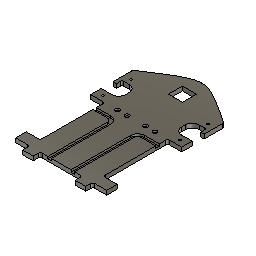
2023_2024_3DP_07.03_Robot_follow_line_v3 (Autodesk Fusion 360 design; units mm, degrees)
Autodesk Fusion 360 part; units mm, degrees
note: some values were not read from the file. Set by a fixed rule: the direction of a hole.
sketch "Sketch1" plane through (0, 0, 0) normal (0, 0, 1) x (1, 0, 0)
  line L0 (-65, -210) -> (-48, -210)
  line L1 (-45, -213) -> (-45, -220)
  line L2 (-45, -220) -> (-30, -220)
  line L3 (-30, -220) -> (-30, -213)
  line L4 (-27, -210) -> (0, -210)
  arc A0 (-45, -213) -> (-48, -210) centre (-48, -213) ccw
  arc A1 (-27, -210) -> (-30, -213) centre (-27, -213) ccw
  line L5 (-65, -210) -> (-65, -195)
  line L6 (-65, -195) -> (-48, -195)
  line L7 (-45, -192) -> (-45, -106)
  line L8 (-48, -103) -> (-65, -103)
  line L9 (-65, -103) -> (-65, -88)
  line L10 (-65, -88) -> (-50, -88)
  line L11 (-40, -78) -> (-40, -73)
  line L12 (-65, -63) -> (-65, -44.6163)
  arc A2 (-50, -88) -> (-40, -78) centre (-50, -78) ccw
  arc A3 (-40, -73) -> (-50, -63) centre (-50, -73) ccw
  arc A4 (-48, -195) -> (-45, -192) centre (-48, -192) ccw
  arc A5 (-45, -106) -> (-48, -103) centre (-48, -106) ccw
  line L13 (-65, -63) -> (-65, -71)
  line L14 (-65, -71) -> (-60, -71)
  line L15 (-60, -71) -> (-60, -65)
  line L16 (-58, -63) -> (-50, -63)
  arc A6 (-58, -63) -> (-60, -65) centre (-58, -65) ccw
  line L17 (-63.6502, -42.1109) -> (-56.6488, -37.4994)
  arc A7 (-63.6502, -42.1109) -> (-65, -44.6163) centre (-62, -44.6163) ccw
  line L18 (0, 0) -> (0, -252.3978) construction
  spline S0 degree 2 poles (-56.6488, -37.4994) (-14.1632, -9.3755) (0, -9.5) knots 0 0 0 6.369294 6.369294 6.369294 weights 1 1.414179 1
  line L19 (-10, -27) -> (0, -27)
  line L20 (0, -47) -> (-10, -47)
  line L21 (-10, -47) -> (-10, -27)
  circle A8 centre (-13, -103) radius 3
  circle A9 centre (-27, -103) radius 3
  line L22 (-13, -103) -> (-27, -103)
  line L23 (45, -220) -> (30, -220)
  line L24 (63.6502, -42.1109) -> (56.6488, -37.4994)
  line L25 (65, -210) -> (48, -210)
  line L26 (45, -192) -> (45, -106)
  line L27 (58, -63) -> (50, -63)
  line L28 (65, -88) -> (50, -88)
  line L29 (0, -47) -> (10, -47)
  line L30 (65, -71) -> (60, -71)
  arc A10 (48, -210) -> (45, -213) centre (48, -213) ccw
  line L31 (48, -103) -> (65, -103)
  arc A11 (50, -63) -> (40, -73) centre (50, -73) ccw
  line L32 (10, -27) -> (0, -27)
  line L33 (65, -63) -> (65, -71)
  line L34 (40, -78) -> (40, -73)
  arc A12 (60, -65) -> (58, -63) centre (58, -65) ccw
  line L35 (60, -71) -> (60, -65)
  spline S1 degree 2 poles (56.6488, -37.4994) (14.1632, -9.3755) (0, -9.5) knots 0 0 0 6.369294 6.369294 6.369294 weights 1 1.414179 1
  line L36 (65, -63) -> (65, -44.6163)
  circle A13 centre (27, -103) radius 3
  arc A14 (30, -213) -> (27, -210) centre (27, -213) ccw
  line L37 (13, -103) -> (27, -103)
  arc A15 (65, -44.6163) -> (63.6502, -42.1109) centre (62, -44.6163) ccw
  arc A16 (45, -192) -> (48, -195) centre (48, -192) ccw
  line L38 (65, -103) -> (65, -88)
  line L39 (30, -220) -> (30, -213)
  arc A17 (40, -78) -> (50, -88) centre (50, -78) ccw
  line L40 (27, -210) -> (0, -210)
  line L41 (10, -47) -> (10, -27)
  line L42 (45, -213) -> (45, -220)
  arc A18 (48, -103) -> (45, -106) centre (48, -106) ccw
  line L43 (65, -195) -> (48, -195)
  line L44 (65, -210) -> (65, -195)
  circle A19 centre (13, -103) radius 3
  point P0 (-45, -210)
  point P1 (-30, -210)
  point P2 (-45, -195)
  point P3 (-45, -103)
  point P4 (-40, -88)
  point P5 (-40, -63)
  point P6 (40, -63)
  point P7 (45, -103)
  point P8 (30, -210)
  point P9 (45, -195)
  point P10 (40, -88)
  point P11 (45, -210)
  dimension "d1" = 20
  dimension "d3" = 15
  dimension "d7" = 3
  dimension "d8" = 3
  dimension "d13" = 20
  dimension "d15" = 92
  dimension "d16" = 15
  dimension "d17" = 25
  dimension "d18" = 25
  dimension "d24" = 10
  dimension "d25" = 10
  dimension "d28" = 3
  dimension "d29" = 3
  dimension "d32" = 5
  dimension "d33" = 2
  dimension "d38" = 3
  dimension "d542" = 10
  dimension "d543" = 9.5
  dimension "d544" = 27
  dimension "d545" = 20
  dimension "d546" = 65
  dimension "d547" = 10
  dimension "d548" = 210
  dimension "d549" = 15
  dimension "d550" = 65
  dimension "d551" = 17
  dimension "d552" = 8
  dimension "d553" = 6
  dimension "d554" = 6
  dimension "d555" = 13
  dimension "d556" = 14
  constraint horizontal L0
  constraint perpendicular L0 L1
  constraint perpendicular L1 L2
  constraint perpendicular L2 L3
  constraint perpendicular L3 L4
  constraint coincident P0 L0
  constraint coincident P0 L1
  constraint tangent L0 A0
  constraint tangent L1 A0
  constraint coincident P1 L3
  constraint coincident P1 L4
  constraint tangent L3 A1
  constraint tangent L4 A1
  constraint perpendicular L0 L5
  constraint perpendicular L5 L6
  constraint perpendicular L6 L7
  constraint perpendicular L7 L8
  constraint perpendicular L8 L9
  constraint perpendicular L7 L10
  constraint perpendicular L8 L11
  constraint coincident P4 L10
  constraint coincident P4 L11
  constraint tangent L10 A2
  constraint tangent L11 A2
  constraint coincident P5 L11
  constraint tangent L11 A3
  constraint coincident P2 L6
  constraint coincident P2 L7
  constraint tangent L6 A4
  constraint tangent L7 A4
  constraint coincident P3 L7
  constraint coincident P3 L8
  constraint tangent L7 A5
  constraint tangent L8 A5
  constraint parallel L12 L13
  constraint perpendicular L13 L14
  constraint perpendicular L14 L15
  constraint tangent A3 L16
  constraint tangent L16 A6
  constraint tangent L15 A6
  constraint tangent L12 A7
  constraint tangent L17 A7
  constraint coincident L18.start origin
  constraint parallel L7 L18
  constraint coincident L18 S0.end
  constraint coincident L18 L4.end
  constraint horizontal L19
  constraint horizontal L20
  constraint vertical L21
  constraint coincident L18 L19.end
  constraint coincident L18 L20.start
  constraint collinear L0 L4
  constraint collinear L9 L12
  constraint coincident A8.centre L22.start
  constraint coincident A9.centre L22.end
  constraint horizontal L22
  constraint collinear L8 L22
  constraint symmetric L0.start L18 L25.start
  constraint symmetric P0 L18 P11
  constraint symmetric L1.end L18 L23.start
  constraint symmetric L2.end L18 L23.end
  constraint symmetric P1 L18 P8
  constraint symmetric L0.end L18 L25.end
  constraint symmetric L1.start L18 A10.end
  constraint symmetric A0 L18 A10
  constraint symmetric L3.end L18 A14.start
  constraint symmetric L4.start L18 A14.end
  constraint symmetric A1 L18 A14
  constraint symmetric L5.end L18 L43.start
  constraint symmetric P2 L18 P9
  constraint symmetric P3 L18 P7
  constraint symmetric L8.end L18 L31.end
  constraint symmetric L9.end L18 L28.start
  constraint symmetric P4 L18 P10
  constraint symmetric P5 L18 P6
  constraint symmetric L12.start L18 L33.start
  constraint symmetric L10.end L18 L28.end
  constraint symmetric L11.start L18 L34.start
  constraint symmetric A2 L18 A17
  constraint symmetric L11.end L18 A11.end
  constraint symmetric A3.end L18 L27.end
  constraint symmetric A3 L18 A11
  constraint symmetric L6.end L18 A16.end
  constraint symmetric L7.start L18 L26.start
  constraint symmetric A4 L18 A16
  constraint symmetric L7.end L18 L26.end
  constraint symmetric L8.start L18 L31.start
  constraint symmetric A5 L18 A18
  constraint symmetric L13.end L18 L30.start
  constraint symmetric L14.end L18 L30.end
  constraint symmetric L16.start L18 L27.start
  constraint symmetric L15.end L18 A12.start
  constraint symmetric A6 L18 A12
  constraint symmetric L17.end L18 L24.end
  constraint symmetric L12.end L18 L36.end
  constraint symmetric L17.start L18 L24.start
  constraint symmetric A7 L18 A15
  constraint symmetric L18 S0.end S1.end
  constraint symmetric L18 S0 S1
  constraint symmetric L18 L4.end L40.end
  constraint symmetric L18 L19.start L32.start
  constraint symmetric L18 L20.end L29.end
  constraint symmetric L18 L19.end L32.end
  constraint symmetric L18 L20.start L29.start
  constraint symmetric L18 A8 A19
  constraint symmetric L18 A9 A13
  constraint symmetric L18 A8.centre L37.start
  constraint symmetric L18 A9.centre A13.centre
  measures "d1" distance of L0.start P0
  measures "d3" distance of L1.end L2.end
  measures "d7" radius of A0
  measures "d8" radius of A1
  measures "d13" distance of L5.end P2
  measures "d15" distance of P2 P3
  measures "d16" distance of L8.end L9.end
  measures "d17" distance of L9.end P4
  measures "d18" distance of P4 P5
  measures "d24" radius of A2
  measures "d25" radius of A3
  measures "d28" radius of A4
  measures "d29" radius of A5
  measures "d32" distance of L13.end L14.end
  measures "d33" radius of A6
  measures "d38" radius of A7
  measures "d542" distance of L19.start L19.end
  measures "d543" distance of L18.start S0.end
  measures "d544" distance of L18.start L19
  measures "d545" distance of L19 L20
  measures "d546" distance of L5 L18
  measures "d547" distance of L2 L4
  measures "d548" distance of L18.start L4
  measures "d549" distance of L0 L6
  measures "d550" distance of L9 L18
  measures "d551" distance of L10 L14
  measures "d552" distance of L14 L16
  measures "d553" diameter of A8
  measures "d554" diameter of A9
  measures "d555" distance of L18 A8.centre
  measures "d556" distance of A8.centre A9.centre
extrude "Extrude8" add sketch "Sketch1" along normal blind 6 contours L0 L1 L2 L3 L4 A0 A1 L5 L6 L7 L8 L9 L10 L11 L12 A2 A3 A4 A5 L13 L14 L15 L16 A6 L17 A7 S0 L23 L24 L25 L26 L27 L28 L30 A10 L31 A11 L33 L34 A12 L35 S1 L36 A14 A15 A16 L38 L39 A17 L40 L42 A18 L43 L44 | A8 | A9 | A13 | A19
sketch "Sketch7" plane through (0, 0, 6) normal (0, 0, 1) x (-1, 0, 0)
  line L0 (-10, 47) -> (10, 47)
  line L1 (10, 47) -> (10, 27)
  line L2 (10, 27) -> (-10, 27)
  line L3 (-10, 27) -> (-10, 47)
  line L4 (-48, 210) -> (-65, 210)
  line L5 (-65, 210) -> (-65, 195)
  line L6 (-65, 195) -> (-48, 195)
  arc A0 (-45, 192) -> (-48, 195) centre (-48, 192) ccw
  line L7 (-45, 192) -> (-45, 106)
  arc A1 (-48, 103) -> (-45, 106) centre (-48, 106) ccw
  line L8 (-48, 103) -> (-65, 103)
  line L9 (-65, 103) -> (-65, 88)
  line L10 (-65, 88) -> (-50, 88)
  arc A2 (-40, 78) -> (-50, 88) centre (-50, 78) ccw
  line L11 (-40, 78) -> (-40, 73)
  arc A3 (-50, 63) -> (-40, 73) centre (-50, 73) ccw
  line L12 (-50, 63) -> (-58, 63)
  arc A4 (-60, 65) -> (-58, 63) centre (-58, 65) ccw
  line L13 (-60, 65) -> (-60, 71)
  line L14 (-60, 71) -> (-65, 71)
  line L15 (-65, 71) -> (-65, 44.6163)
  arc A5 (-65, 44.6163) -> (-63.6502, 42.1109) centre (-62, 44.6163) ccw
  line L16 (-63.6502, 42.1109) -> (-56.6488, 37.4994)
  spline S0 degree 2 poles (-56.6488, 37.4994) (-14.1632, 9.3755) (0, 9.5) knots 0 0 0 6.369294 6.369294 6.369294 weights 1 1.414179 1
  spline S1 degree 2 poles (0, 9.5) (14.1632, 9.3755) (56.6488, 37.4994) knots -6.369294 -6.369294 -6.369294 0 0 0 weights 1 1.414179 1
  line L17 (56.6488, 37.4994) -> (63.6502, 42.1109)
  arc A6 (63.6502, 42.1109) -> (65, 44.6163) centre (62, 44.6163) ccw
  line L18 (65, 44.6163) -> (65, 71)
  line L19 (65, 71) -> (60, 71)
  line L20 (60, 71) -> (60, 65)
  arc A7 (58, 63) -> (60, 65) centre (58, 65) ccw
  line L21 (58, 63) -> (50, 63)
  arc A8 (40, 73) -> (50, 63) centre (50, 73) ccw
  line L22 (40, 73) -> (40, 78)
  arc A9 (50, 88) -> (40, 78) centre (50, 78) ccw
  line L23 (50, 88) -> (65, 88)
  line L24 (65, 88) -> (65, 103)
  line L25 (65, 103) -> (48, 103)
  arc A10 (45, 106) -> (48, 103) centre (48, 106) ccw
  line L26 (45, 106) -> (45, 192)
  arc A11 (48, 195) -> (45, 192) centre (48, 192) ccw
  line L27 (48, 195) -> (65, 195)
  line L28 (65, 195) -> (65, 210)
  line L29 (65, 210) -> (48, 210)
  arc A12 (45, 213) -> (48, 210) centre (48, 213) ccw
  line L30 (45, 213) -> (45, 220)
  line L31 (45, 220) -> (30, 220)
  line L32 (30, 220) -> (30, 213)
  arc A13 (27, 210) -> (30, 213) centre (27, 213) ccw
  line L33 (27, 210) -> (-27, 210)
  arc A14 (-30, 213) -> (-27, 210) centre (-27, 213) ccw
  line L34 (-30, 213) -> (-30, 220)
  line L35 (-30, 220) -> (-45, 220)
  line L36 (-45, 220) -> (-45, 213)
  arc A15 (-48, 210) -> (-45, 213) centre (-48, 213) ccw
  circle A16 centre (27, 103) radius 3
  circle A17 centre (13, 103) radius 3
  circle A18 centre (-13, 103) radius 3
  circle A19 centre (-27, 103) radius 3
  line L37 (0, 0) -> (0, 252.3978)
  line L38 (-13, 103) -> (-27, 103)
  line L39 (13, 103) -> (27, 103)
  point P0 (27, 103)
  point P1 (13, 103)
  point P2 (-13, 103)
  point P3 (-27, 103)
hole "Hole1" at (-27, -103, 0) at (-13, -103, 0) at (13, -103, 0) at (27, -103, 0) direction (0, 0, 1) diameter 10 depth 3 tip angle 180
extrude "Extrude9" cut sketch "Sketch7" against normal blind 2.5 contours A16 | A17 | A18 | A19
sketch "Sketch8" plane through (0, 0, 6) normal (0, 0, 1) x (-1, 0, 0)
  circle A0 centre (13, 103) radius 3
  circle A1 centre (-13, 103) radius 3
  circle A2 centre (27, 103) radius 3
  circle A3 centre (-27, 103) radius 3
  line L0 (-10, 47) -> (10, 47)
  line L1 (10, 47) -> (10, 27)
  line L2 (10, 27) -> (-10, 27)
  line L3 (-10, 27) -> (-10, 47)
  line L4 (-48, 210) -> (-65, 210)
  line L5 (-65, 210) -> (-65, 195)
  line L6 (-65, 195) -> (-48, 195)
  arc A4 (-45, 192) -> (-48, 195) centre (-48, 192) ccw
  line L7 (-45, 192) -> (-45, 106)
  arc A5 (-48, 103) -> (-45, 106) centre (-48, 106) ccw
  line L8 (-48, 103) -> (-65, 103)
  line L9 (-65, 103) -> (-65, 88)
  line L10 (-65, 88) -> (-50, 88)
  arc A6 (-40, 78) -> (-50, 88) centre (-50, 78) ccw
  line L11 (-40, 78) -> (-40, 73)
  arc A7 (-50, 63) -> (-40, 73) centre (-50, 73) ccw
  line L12 (-50, 63) -> (-58, 63)
  arc A8 (-60, 65) -> (-58, 63) centre (-58, 65) ccw
  line L13 (-60, 65) -> (-60, 71)
  line L14 (-60, 71) -> (-65, 71)
  line L15 (-65, 71) -> (-65, 44.6163)
  arc A9 (-65, 44.6163) -> (-63.6502, 42.1109) centre (-62, 44.6163) ccw
  line L16 (-63.6502, 42.1109) -> (-56.6488, 37.4994)
  spline S0 degree 2 poles (-56.6488, 37.4994) (-14.1632, 9.3755) (0, 9.5) knots 0 0 0 6.369294 6.369294 6.369294 weights 1 1.414179 1
  spline S1 degree 2 poles (0, 9.5) (14.1632, 9.3755) (56.6488, 37.4994) knots -6.369294 -6.369294 -6.369294 0 0 0 weights 1 1.414179 1
  line L17 (56.6488, 37.4994) -> (63.6502, 42.1109)
  arc A10 (63.6502, 42.1109) -> (65, 44.6163) centre (62, 44.6163) ccw
  line L18 (65, 44.6163) -> (65, 71)
  line L19 (65, 71) -> (60, 71)
  line L20 (60, 71) -> (60, 65)
  arc A11 (58, 63) -> (60, 65) centre (58, 65) ccw
  line L21 (58, 63) -> (50, 63)
  arc A12 (40, 73) -> (50, 63) centre (50, 73) ccw
  line L22 (40, 73) -> (40, 78)
  arc A13 (50, 88) -> (40, 78) centre (50, 78) ccw
  line L23 (50, 88) -> (65, 88)
  line L24 (65, 88) -> (65, 103)
  line L25 (65, 103) -> (48, 103)
  arc A14 (45, 106) -> (48, 103) centre (48, 106) ccw
  line L26 (45, 106) -> (45, 192)
  arc A15 (48, 195) -> (45, 192) centre (48, 192) ccw
  line L27 (48, 195) -> (65, 195)
  line L28 (65, 195) -> (65, 210)
  line L29 (65, 210) -> (48, 210)
  arc A16 (45, 213) -> (48, 210) centre (48, 213) ccw
  line L30 (45, 213) -> (45, 220)
  line L31 (45, 220) -> (30, 220)
  line L32 (30, 220) -> (30, 213)
  arc A17 (27, 210) -> (30, 213) centre (27, 213) ccw
  line L33 (27, 210) -> (-27, 210)
  arc A18 (-30, 213) -> (-27, 210) centre (-27, 213) ccw
  line L34 (-30, 213) -> (-30, 220)
  line L35 (-30, 220) -> (-45, 220)
  line L36 (-45, 220) -> (-45, 213)
  arc A19 (-48, 210) -> (-45, 213) centre (-48, 213) ccw
  line L37 (0, 0) -> (0, 252.3978)
  line L38 (45, 192) -> (45, 106)
  line L39 (27, 210) -> (0, 210)
  line L40 (45, 115) -> (24, 115)
  line L41 (11.7685, 115) -> (11.7685, 119.6256)
  line L42 (18, 111.5381) -> (14, 111.5381)
  line L43 (14, 125) -> (14, 210)
  arc A20 (14, 125) -> (24, 115) centre (24, 125) ccw
  line L44 (45, 120) -> (24, 120)
  arc A21 (19, 125) -> (24, 120) centre (24, 125) ccw
  line L45 (19, 125) -> (19, 210)
  line L46 (45, 115) -> (45, 120)
  line L47 (14, 210) -> (19, 210)
  line L48 (-18, 111.5381) -> (-14, 111.5381)
  line L49 (-14, 125) -> (-14, 210)
  line L50 (-11.7685, 115) -> (-11.7685, 119.6256)
  line L51 (-45, 115) -> (-24, 115)
  line L52 (-45, 120) -> (-24, 120)
  arc A22 (-24, 120) -> (-19, 125) centre (-24, 125) ccw
  arc A23 (-24, 115) -> (-14, 125) centre (-24, 125) ccw
  line L53 (-19, 125) -> (-19, 210)
  line L54 (-45, 115) -> (-45, 120)
  line L55 (-14, 210) -> (-19, 210)
  dimension "d564" = 14
  dimension "d567" = 10
  dimension "d568" = 95
  dimension "d569" = 5
  constraint horizontal L40
  constraint vertical L41
  constraint horizontal L42
  constraint vertical L43
  constraint coincident L33 L43.end
  constraint coincident L41.start L40
  constraint coincident L42.end L43
  constraint tangent L40 A20
  constraint tangent L43 A20
  constraint coincident L26 L40.start
  constraint symmetric L37 L41.start L50.start
  constraint symmetric L37 L41.end L50.end
  constraint symmetric L37 L42.start L48.start
  constraint symmetric L37 L42.end L48.end
  constraint symmetric L37 L43.end L49.end
  constraint symmetric L37 L40.end L51.end
  constraint symmetric L37 L43.start L49.start
  constraint symmetric L37 A20 A23
  constraint symmetric L37 L40.start L51.start
  constraint symmetric L37 L44.start L52.start
  constraint symmetric L37 L44.end L52.end
  constraint symmetric L37 A21.start A22.end
  constraint symmetric L37 A21 A22
  constraint symmetric L37 L45.end L53.end
  measures "d564" distance of L37 L43
  measures "d567" radius of A20
  measures "d568" distance of L39 L40
extrude "Extrude10" cut sketch "Sketch8" against normal blind 3 contours L26 L33 L38 L39 L40 L43 A20 L44 A21 L45 L46 L47 | L7 L33 L49 L51 L52 A22 A23 L53 L54 L55
sketch "Sketch9" plane through (0, 0, 6) normal (0, 0, 1) x (-1, 0, 0)
  line L0 (45, 115) -> (24, 115)
  arc A0 (14, 125) -> (24, 115) centre (24, 125) ccw
  line L1 (14, 125) -> (14, 210)
  line L2 (14, 210) -> (-14, 210)
  line L3 (-14, 210) -> (-14, 125)
  arc A1 (-24, 115) -> (-14, 125) centre (-24, 125) ccw
  line L4 (-24, 115) -> (-45, 115)
  line L5 (-45, 115) -> (-45, 106)
  arc A2 (-48, 103) -> (-45, 106) centre (-48, 106) ccw
  line L6 (-48, 103) -> (-65, 103)
  line L7 (-65, 103) -> (-65, 88)
  line L8 (-65, 88) -> (-50, 88)
  arc A3 (-40, 78) -> (-50, 88) centre (-50, 78) ccw
  line L9 (-40, 78) -> (-40, 73)
  arc A4 (-50, 63) -> (-40, 73) centre (-50, 73) ccw
  line L10 (-50, 63) -> (-58, 63)
  arc A5 (-60, 65) -> (-58, 63) centre (-58, 65) ccw
  line L11 (-60, 65) -> (-60, 71)
  line L12 (-60, 71) -> (-65, 71)
  line L13 (-65, 71) -> (-65, 44.6163)
  arc A6 (-65, 44.6163) -> (-63.6502, 42.1109) centre (-62, 44.6163) ccw
  line L14 (-63.6502, 42.1109) -> (-56.6488, 37.4994)
  spline S0 degree 2 poles (-56.6488, 37.4994) (-14.1632, 9.3755) (0, 9.5) knots 0 0 0 6.369294 6.369294 6.369294 weights 1 1.414179 1
  spline S1 degree 2 poles (0, 9.5) (14.1632, 9.3755) (56.6488, 37.4994) knots -6.369294 -6.369294 -6.369294 0 0 0 weights 1 1.414179 1
  line L15 (56.6488, 37.4994) -> (63.6502, 42.1109)
  arc A7 (63.6502, 42.1109) -> (65, 44.6163) centre (62, 44.6163) ccw
  line L16 (65, 44.6163) -> (65, 71)
  line L17 (65, 71) -> (60, 71)
  line L18 (60, 71) -> (60, 65)
  arc A8 (58, 63) -> (60, 65) centre (58, 65) ccw
  line L19 (58, 63) -> (50, 63)
  arc A9 (40, 73) -> (50, 63) centre (50, 73) ccw
  line L20 (40, 73) -> (40, 78)
  arc A10 (50, 88) -> (40, 78) centre (50, 78) ccw
  line L21 (50, 88) -> (65, 88)
  line L22 (65, 88) -> (65, 103)
  line L23 (65, 103) -> (48, 103)
  arc A11 (45, 106) -> (48, 103) centre (48, 106) ccw
  line L24 (45, 106) -> (45, 115)
  line L25 (-10, 47) -> (10, 47)
  line L26 (10, 47) -> (10, 27)
  line L27 (10, 27) -> (-10, 27)
  line L28 (-10, 27) -> (-10, 47)
  circle A12 centre (-27, 103) radius 3
  circle A13 centre (27, 103) radius 3
  circle A14 centre (-13, 103) radius 3
  circle A15 centre (13, 103) radius 3
  line L29 (74.2747, 95.5) -> (35.7253, 95.5)
  circle A16 centre (55, 95.5) radius 1
  line L30 (40, 75.5) -> (74.2747, 75.5)
  circle A17 centre (55, 55.5) radius 1
  line L31 (0, 0) -> (0, 252.3978)
  point P0 (-55, 55.5)
  point P1 (-55, 95.5)
  dimension "d572" = 2
  dimension "d573" = 10
  constraint perpendicular L22 L29
  constraint midpoint L29 A16.centre
  constraint midpoint L20 L30.start
  constraint perpendicular L20 L30
  constraint symmetric A16 L30 A17
  constraint symmetric A16.centre L31 P1
  constraint symmetric A17.centre L31 P0
  measures "d572" diameter of A16
  measures "d573" distance of L22 A16.centre
hole "Hole2" at (55, -55.5, 6) at (55, -95.5, 6) at (-55, -95.5, 6) at (-55, -55.5, 6) direction (0, 0, -1) diameter 3 end through all
